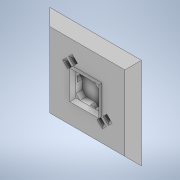
# Autodesk Inventor part: clear-square-reed
Saved by Autodesk Inventor 2021 (Build 250183000, 183)
## iProperties
Created: 2020-12-08
Part Number: clear-square-reed
Material: Generic
Document SubType Name: Modeling
Designer: Luke Kamols
Density: 1 g/cm^3
Appearance: Default
Author: Luke Kamols
Autodesk Inventor part; units mm, degrees
ref_plane "YZ Plane" through (0, 0, 0) normal (1, 0, 0) x (0, 1, 0)
sketch "Sketch1" plane through (0, 0, 0) normal (0, 0, 1) x (1, 0, 0)
  line L0 (0, 0) -> (44, 0)
  line L1 (44, 0) -> (44, 44)
  line L2 (44, 44) -> (0, 44)
  line L3 (0, 44) -> (0, 0)
  dimension "d0" = 44
  dimension "d1" = 44
  constraints: 8 end point, 2 parallel, 1 horizontal, 1 perpendicular
  measures "d0" distance of L2.end L1.end
  measures "d1" distance of L1.end L0.end
extrude "Extrusion1" add sketch "Sketch1" along normal blind 4
chamfer "Chamfer1" distance 4 angle 45 4 edges at (22, 44, 4) (44, 22, 4) (22, 0, 4) (0, 22, 4)
sketch "Sketch2" plane through (0, 0, 4) normal (0, 0, 1) x (1, 0, 0)
  line L0 (40, 4) -> (4, 4) projected
  line L1 (40, 40) -> (40, 4) projected
  line L2 (4, 40) -> (40, 40) projected
  line L3 (4, 4) -> (4, 40) projected
  line L4 (40, 4) -> (4, 4) projected
  line L5 (40, 40) -> (40, 4) projected
  line L6 (4, 4) -> (40, 40)
  line L7 (4, 40) -> (40, 40) projected
  line L8 (40, 4) -> (4, 40)
  line L9 (22, 16.5) -> (16.5, 16.5)
  line L10 (16.5, 16.5) -> (16.5, 27.5)
  line L11 (16.5, 27.5) -> (27.5, 27.5)
  line L12 (27.5, 27.5) -> (27.5, 16.5)
  line L13 (27.5, 16.5) -> (22, 16.5)
  line L14 (27.5, 27.5) -> (27.5, 25.5)
  arc A0 (18.5, 27.5) -> (16.5, 25.5) centre (18.5, 25.5) ccw
  line L15 (18.5, 25.5) -> (18.5, 18.5)
  line L16 (18.5, 18.5) -> (25.5, 18.5)
  line L17 (25.5, 18.5) -> (25.5, 25.5)
  arc A1 (16.5, 18.5) -> (18.5, 16.5) centre (18.5, 18.5) ccw
  arc A2 (25.5, 16.5) -> (27.5, 18.5) centre (25.5, 18.5) ccw
  arc A3 (27.5, 25.5) -> (25.5, 27.5) centre (25.5, 25.5) ccw
  line L18 (27.5, 18.5) -> (25.5, 16.5)
  line L19 (18.5, 16.5) -> (16.5, 18.5)
  line L20 (16.5, 25.5) -> (18.5, 27.5)
  line L21 (25.5, 27.5) -> (27.5, 25.5)
  point P0 (0, 0)
  dimension "d86" = 2
  constraints: 30 end point, 16 point on line, 8 point on circle, 4 centre point, 4 tangent, 3 coincident, 3 perpendicular
  measures "d86" distance of L14.end L11.end
extrude "Extrusion2" cut sketch "Sketch2" against normal blind 3 contours L18 L8 L17 L6 L21 L12 | L13 L9 L19 L6 L16 L8 L18 | L10 L20 L8 L15 L6 L19 | L21 L6 L8 L20 L11 | L16 L6 L8 | L8 L6 L17 | L15 L8 L6
ref_plane "Work Plane3" through (27.5, 16.5, 4) normal (-0.7071, -0.7071, 0) x (0, 0, 1)
ref_plane "Work Plane4" through (27.5, 27.5, 4) normal (0.7071, -0.7071, 0) x (0, 0, 1)
ref_plane "Work Plane5" through (26.0858, 15.0858, 4) normal (-0.7071, -0.7071, 0) x (0, 0, 1)
sketch "Sketch13" plane through (27.5, 27.5, 4) normal (0.7071, -0.7071, 0) x (0, 0, 1)
  line L0 (-4.8, 9.7782) -> (0.8, 9.7782) projected
  line L1 (-3, 9.1924) -> (-3, 14.1421) projected
  line L2 (-3, 9.7782) -> (-3, 11.0282)
  line L3 (-3, 11.0282) -> (-0.5, 11.0282)
  line L4 (-0.5, 11.0282) -> (-0.5, 8.5282)
  line L5 (-0.5, 8.5282) -> (-3, 8.5282)
  line L6 (-3, 8.5282) -> (-3, 9.7782)
  point P0 (-4, 38.8909)
  point P1 (-3, 9.1924)
  dimension "d88" = 1.25
  dimension "d89" = 2.5
  dimension "d90" = 2.5
  constraints: 10 end point, 4 point on line, 3 perpendicular, 1 collinear
  measures "d88" distance of L2.start L2.end
  measures "d89" distance of L2.end L3.end
  measures "d90" distance of L3.end L4.end
sketch "Sketch14" plane through (26.0858, 15.0858, 4) normal (-0.7071, -0.7071, 0) x (0, 0, 1)
  line L0 (-3, 7.7782) -> (-1.75, 7.7782)
  line L1 (-1.75, 7.7782) -> (-1.75, 17.7782)
  line L2 (-1.75, 17.7782) -> (0, 19.5282)
  line L3 (-1.75, 17.7782) -> (0.7249, 17.7782) construction
  line L4 (-1.75, 7.7782) -> (-1.75, -2.2218)
  line L5 (-1.75, -2.2218) -> (0, -3.9718)
  line L6 (0, 19.5282) -> (2.0141, 21.5422)
  line L7 (0, -3.9718) -> (2.0141, -5.9859)
  point P0 (-4, 7.7782)
  dimension "d91" = 1.25
  dimension "d92" = 10
  dimension "d93" = 45
  dimension "d94" = 10
  constraints: 16 end point, 2 horizontal, 2 vertical, 1 equal length
  measures "d91" distance of L0.start L0.end
  measures "d92" distance of L0.end L1.end
  measures "d93" angle of L3 L2
  measures "d94" distance of L0.end L4.end
sweep "Sweep3" cut profiles "Sketch13" path "Sketch14" path curves L7 L5 L4 L1 L2 L6
mirror "Mirror2" about plane through (27.5, 16.5, 4) normal (-0.7071, -0.7071, 0) of "Sweep3"
sketch "Sketch15" plane through (0, 0, 4) normal (0, 0, 1) x (1, 0, 0)
  line L0 (17.2396, 31.3566) -> (15.4718, 29.5888) projected
  line L1 (15.4718, 29.5888) -> (12.9718, 32.0888) projected
  line L2 (12.9718, 32.0888) -> (14.7396, 33.8566) projected
  line L3 (14.7396, 33.8566) -> (17.2396, 31.3566) projected
  line L4 (31.3566, 17.2396) -> (33.8566, 14.7396) projected
  line L5 (33.8566, 14.7396) -> (32.0888, 12.9718) projected
  line L6 (32.0888, 12.9718) -> (29.5888, 15.4718) projected
  line L7 (29.5888, 15.4718) -> (31.3566, 17.2396) projected
  line L8 (14.4112, 28.5282) -> (12.6434, 26.7604) projected
  line L9 (12.6434, 26.7604) -> (10.1434, 29.2604) projected
  line L10 (10.1434, 29.2604) -> (11.9112, 31.0282) projected
  line L11 (11.9112, 31.0282) -> (14.4112, 28.5282) projected
  line L12 (29.2604, 10.1434) -> (26.7604, 12.6434) projected
  line L13 (26.7604, 12.6434) -> (28.5282, 14.4112) projected
  line L14 (28.5282, 14.4112) -> (31.0282, 11.9112) projected
  line L15 (31.0282, 11.9112) -> (29.2604, 10.1434) projected
  line L16 (18.5, 16.5) -> (16.5, 18.5) projected
  line L17 (16.5, 18.5) -> (16.5, 25.5) projected
  line L18 (16.5, 25.5) -> (18.5, 27.5) projected
  line L19 (18.5, 27.5) -> (25.5, 27.5) projected
  line L20 (25.5, 27.5) -> (27.5, 25.5) projected
  line L21 (27.5, 25.5) -> (27.5, 18.5) projected
  line L22 (27.5, 18.5) -> (25.5, 16.5) projected
  line L23 (25.5, 16.5) -> (18.5, 16.5) projected
  line L24 (40, 4) -> (4, 4) projected
  line L25 (40, 40) -> (40, 4) projected
  line L26 (4, 40) -> (40, 40) projected
  line L27 (4, 4) -> (4, 40) projected
  line L28 (16.5, 18.5) -> (16.5, 22.9038) projected
  line L29 (15, 22.9038) -> (15, 29)
  line L30 (15, 29) -> (29, 29)
  line L31 (29, 29) -> (29, 15)
  line L32 (29, 15) -> (15, 15)
  line L33 (15, 15) -> (15, 29)
  line L34 (16.5, 18.5) -> (16.5, 16.5)
  line L35 (16.5, 16.5) -> (18.5, 16.5)
  line L36 (25.5, 16.5) -> (22.9038, 16.5) projected
  line L37 (25.5, 16.5) -> (27.5, 16.5)
  line L38 (27.5, 16.5) -> (27.5, 18.5)
  line L39 (27.5, 25.5) -> (27.5, 27.5)
  line L40 (25.5, 27.5) -> (27.5, 25.5) projected
  line L41 (27.5, 27.5) -> (25.5, 27.5)
  line L42 (18.5, 27.5) -> (16.5, 27.5)
  line L43 (16.5, 27.5) -> (16.5, 25.5)
  point P0 (0, 0)
  dimension "d97" = 1.5
  constraints: 26 end point, 6 perpendicular, 5 point on line, 2 vertical, 1 horizontal
  measures "d97" distance of L28.end L29.start
extrude "Extrusion7" add sketch "Sketch15" along normal blind 1.5 contours L29 L30 L31 L32 L33
chamfer "Chamfer6" distance 1.5 angle 45 4 edges at (22, 16.5, 5.5) (16.5, 22, 5.5) (27.5, 22, 5.5) (22, 27.5, 5.5)
body "Solid1"
